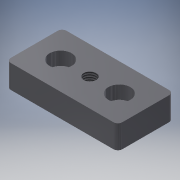
# Autodesk Inventor part: 21-002
Saved by Autodesk Inventor 2018 (Build 220105000, 105)
## iProperties
Created: 2004-10-15
Part Number: 21-002
Material: Steel, High Strength Low Alloy
Document SubType Name: Modeling
Designer: Autodesk, Inc.
Manufacturer: Standard
Standards Organization: Custom
Description: BASE PLATE, 40 SERIES, 40x80, M10
Vendor: PARKER IPS
Catalog Web Link: http://www.parker.com/ead/cm1.asp?cmid=809
Mass: 320.354 g
Surface Area: 105.96 cm^2
Volume: 40.8615 cm^3
Density: 7.84 g/cm^3
Appearance: Metal-Steel (Polished)
CAGE: 1LJX3
Dept. ID: Product Design
Description #2: ---
Finish #1: ---
Finish #2: ---
Material ID: ---
Project Number: ---
Author: Autodesk, Inc.
Autodesk Inventor part; units mm, degrees
ref_plane "YZ Plane" through (0, 0, 0) normal (1, 0, 0) x (0, 1, 0)
ref_plane "XZ Plane" through (0, 0, 0) normal (0, 1, 0) x (-1, 0, 0)
ref_plane "XY Plane" through (0, 0, 0) normal (0, 0, 1) x (1, 0, 0)
sketch "Sketch1" plane through (0, 0, 0) normal (0, 0, 1) x (1, 0, 0)
  line L0 (-38, 19) -> (38, 19)
  line L1 (38, 19) -> (38, -19)
  line L2 (38, -19) -> (-38, -19)
  line L3 (-38, -19) -> (-38, 19)
  point P0 (0, 0)
  point P1 (0, 19)
  point P2 (-38, 0)
  dimension "Dim_A" = 76
  dimension "Dim_B" = 38
  constraints: 8 end point, 2 midpoint, 2 parallel, 1 horizontal, 1 horizontal alignment, 1 perpendicular, 1 vertical alignment
  measures "Dim_A" distance of L1.end L2.end
  measures "Dim_B" distance of L0.end L1.end
extrude "Base" add sketch "Sketch1" against normal mid plane 15.9
sketch "Sketch2" plane through (0, 0, 7.95) normal (0, 0, 1) x (1, 0, 0)
  line L0 (0, -26.6) -> (0, 26.6) construction
  line L1 (-53.2, 0) -> (53.2, 0) construction
  point P0 (0, 0)
  point P1 (0, 0)
  point P2 (-20, 0)
  dimension "Dim_D1" = 0
  dimension "Dim_D" = 40
  constraints: 1 coincident
  measures "Dim_D1" distance from line of point (-20, 0) L1
  measures "Dim_D" diameter of point (-20, 0) L0
hole "MountHole" at (-20, 0, 7.95) direction (0, 0, -1) diameter 9 end through all counterbore diameter 15 counterbore depth 9
hole "CenterHole" at (0, 0, 7.95) direction (0, 0, -1) diameter 8.376 end through all thread size "M10x1.5" class "6H" standard "ANSI Metric M Profile"
pattern_linear "Mount Hole Pattern" count 2 spacing 40 along (1, 0, 0) of "MountHole"
fillet "Fillet1" radius 3 4 edges at (-38, -19, 0) (-38, 19, 0) (38, 19, 0) (38, -19, 0)
body "Solid1"
